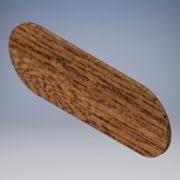
# Autodesk Inventor part: Front Panel
Saved by Autodesk Inventor 2016 SP2 (Build 200236200, 236)
## iProperties
Created: 2017-10-06
Part Number: Front Panel
Material: Wood (Walnut)
Document SubType Name: Modeling
Designer: Jared
Density: 0.55 g/cm^3
Appearance: White Ash - Java
Author: Jared
Autodesk Inventor part; units mm, degrees
ref_plane "YZ Plane" through (0, 0, 0) normal (1, 0, 0) x (0, 1, 0)
ref_plane "XZ Plane" through (0, 0, 0) normal (0, 1, 0) x (-1, 0, 0)
ref_plane "XY Plane" through (0, 0, 0) normal (0, 0, 1) x (1, 0, 0)
sketch "Sketch1" plane through (0, 0, 0) normal (0, 0, 1) x (1, 0, 0)
  line L0 (0, 0) -> (-177.8, 0) construction
  line L1 (0, 50.8) -> (-177.8, 50.8)
  line L2 (-177.8, -50.8) -> (0, -50.8)
  arc A0 (0, -50.8) -> (0, 50.8) centre (0, 0) ccw
  arc A1 (-177.8, 50.8) -> (-177.8, -50.8) centre (-177.8, 0) ccw
  point P0 (-88.9, 0)
  dimension "d0" = 177.8
  dimension "d1" = 101.6
  constraints: 8 end point, 4 point on circle, 4 tangent, 2 centre point, 1 horizontal, 1 midpoint, 1 parallel
  measures "d0" distance of L0.start L0.end
  measures "d1" diameter of A1
extrude "Extrusion1" add sketch "Sketch1" along normal blind 6.35
body "Solid1"
